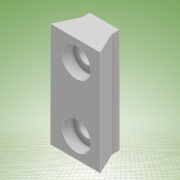
# Autodesk Inventor part: Wall_mount
Saved by Autodesk Inventor 2017 (Build 210142000, 142)
## iProperties
Created: 2018-06-04
Part Number: Wall_mount
Material: Generic
Document SubType Name: Modeling
Designer: Spark Electronics
Density: 1 g/cm^3
Appearance: Default
Author: Spark Electronics
Autodesk Inventor part; units mm, degrees
ref_plane "YZ Plane" through (0, 0, 0) normal (1, 0, 0) x (0, 1, 0)
ref_plane "XZ Plane" through (0, 0, 0) normal (0, 1, 0) x (-1, 0, 0)
ref_plane "XY Plane" through (0, 0, 0) normal (0, 0, 1) x (1, 0, 0)
sketch "Sketch1" plane through (0, 0, 0) normal (0, 0, 1) x (1, 0, 0)
  line L0 (12.6328, -6.7) -> (10.0681, -1.2)
  line L1 (-0.0672, -6.7) -> (2.4975, -1.2)
  line L2 (-0.0672, -6.7) -> (12.6328, -6.7)
  line L3 (10.0681, 0.8) -> (2.4975, 0.8)
  line L4 (2.4975, -1.2) -> (2.4975, 0.8)
  line L5 (10.0681, -1.2) -> (10.0681, 0.8)
  line L6 (2.6975, 0.6) -> (9.8681, 0.6)
  line L7 (9.8681, 0.6) -> (9.8681, -1.2443)
  line L8 (9.8681, -1.2443) -> (12.3189, -6.5)
  line L9 (12.3189, -6.5) -> (0.2468, -6.5)
  line L10 (0.2468, -6.5) -> (2.6975, -1.2443)
  line L11 (2.6975, -1.2443) -> (2.6975, 0.6)
  line L12 (6.2828, 2.7247) -> (6.2828, -9.3147) construction
  point P0 (0, 0)
  point P1 (19.05, 0)
  point P2 (0, 0)
  dimension "d20" = 12.7
  dimension "d22" = 5.5
  dimension "d23" = 5.5
  dimension "d24" = 2
  dimension "d25" = 2
  dimension "d28" = 0.2
  dimension "d29" = 155
  dimension "d31" = 155
  constraints: 26 end point, 2 parallel, 2 perpendicular, 1 horizontal, 1 vertical, 5 other
  measures "d20" distance of L1.start L0.start
  measures "d22" distance from line of L2 L1.end
  measures "d23" distance from line of L2 L0.end
  measures "d24" distance of L1.end L3.end
  measures "d25" distance of L0.end L3.start
  measures "d28" distance between parallel lines of L4 L11
  measures "d29" angle of L1 L4
  measures "d31" angle of L0 L5
extrude "Extrusion1" add sketch "Sketch1" along normal blind 25.4 contours L6 L7 L8 L9 L10 L11
hole "Hole1" at (6.4769, -6.5, 20.4) direction (0, 1, 0) diameter 3.6 end through all counterbore diameter 7 counterbore depth 2.6
hole "Hole2" at (6.4769, -6.5, 5) direction (0, 1, 0) diameter 3.6 end through all counterbore diameter 7 counterbore depth 2.6
body "Solid1"
